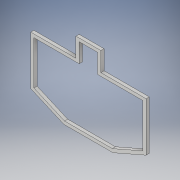
# Autodesk Inventor part: Buste1
Saved by Autodesk Inventor 2018 (Build 220112000, 112)
## iProperties
Created: 2018-02-13
Part Number: Buste1
Material: Generic
Document SubType Name: Modeling
Designer: Lilia
Density: 1 g/cm^3
Appearance: Default
Author: Lilia
Autodesk Inventor part; units mm, degrees
ref_plane "YZ Plane" through (0, 0, 0) normal (1, 0, 0) x (0, 1, 0)
ref_plane "XZ Plane" through (0, 0, 0) normal (0, 1, 0) x (-1, 0, 0)
ref_plane "XY Plane" through (0, 0, 0) normal (0, 0, 1) x (1, 0, 0)
sketch "Sketch1" plane through (0, 0, 0) normal (0, 0, 1) x (1, 0, 0)
  line L0 (107.9, 41.925) -> (107.9, -41.925)
  line L1 (-107.9, -41.925) -> (-107.9, 41.925)
  line L2 (-107.9, 41.925) -> (107.9, -41.925) construction
  line L3 (107.9, 41.925) -> (-107.9, -41.925) construction
  line L4 (-15.6, 80.925) -> (15.6, 80.925)
  line L5 (-15.6, 41.925) -> (-107.9, 41.925)
  line L6 (15.6, 41.925) -> (107.9, 41.925)
  line L7 (-107.9, -41.925) -> (-49.4, -67.398)
  line L8 (107.9, -41.925) -> (49.4, -67.398)
  line L9 (49.4, -67.398) -> (-49.4, -67.398)
  line L10 (-114.4, -47.125) -> (-114.4, 47.125)
  line L11 (114.4, 47.125) -> (114.4, -47.125)
  line L12 (114.4, -47.125) -> (-114.4, 47.125) construction
  line L13 (-114.4, -47.125) -> (114.4, 47.125) construction
  line L14 (-22.1, 47.125) -> (-22.1, 86.125)
  line L15 (-22.1, 86.125) -> (22.1, 86.125)
  line L16 (22.1, 86.125) -> (22.1, 47.125)
  line L17 (22.1, 47.125) -> (114.4, 47.125)
  line L18 (-22.1, 47.125) -> (-114.4, 47.125)
  line L19 (114.4, -47.125) -> (49.4, -75.4283)
  line L20 (-114.4, -47.125) -> (-49.4, -75.4283)
  line L21 (49.4, -75.4283) -> (-49.4, -75.4283)
  line L22 (-15.6, 41.925) -> (-15.6, 80.925)
  line L23 (15.6, 41.925) -> (15.6, 80.925)
  point P0 (0, 0)
  point P1 (0, 0)
  point P2 (0, 80.925)
  point P3 (0, 0)
  point P4 (0, 86.125)
  point P5 (0, 0)
  dimension "Comp" = 215.8
  dimension "Lar" = 83.85
  dimension "Larg1" = 31.2
  dimension "d10" = 215.8
  dimension "d15" = 58.5
  dimension "d16" = 98.8
  dimension "d17" = 58.5
  dimension "LarMaior" = 94.25
  dimension "CompMaior" = 228.8
  dimension "d20" = 39
  dimension "d21" = 44.2
  dimension "d22" = 39
  dimension "d25" = 65
  dimension "d27" = 65
  dimension "d28" = 98.8
  constraints: 48 end point, 9 midpoint, 6 equal length, 3 horizontal, 2 vertical alignment, 1 point on line, 1 vertical
  measures "Comp" distance of L1.end L0.start
  measures "Lar" distance of L1.start L1.end
  measures "Larg1" distance of L4.start L4.end
  measures "d10" distance of L0.end L1.start
  measures "d15" horizontal distance of L0.end L8.end
  measures "d16" distance of L8.end L9.end
  measures "d17" horizontal distance of L1.start L7.end
  measures "LarMaior" distance of L11.start L11.end
  measures "CompMaior" distance of L10.end L11.start
  measures "d20" distance of L15.end L16.end
  measures "d21" distance of L14.end L15.end
  measures "d22" distance of L5.start L4.start
  measures "d25" horizontal distance of L11.end L19.end
  measures "d27" horizontal distance of L10.start L20.end
  measures "d28" distance of L19.end L20.end
extrude "Extrusion1" add sketch "Sketch1" along normal blind 6.5 contours L0 L8 L9 L7 L1 L5 L22 L4 L23 L6 | L10 L18 L14 L15 L16 L17 L11 L19 L21 L20
shell "Shell1" thickness 6.5 both sides yes removed faces 2 at (-7.3667, -34.5772, 6.5) at (-7.3667, -34.5772, 0)
body "Solid1"
